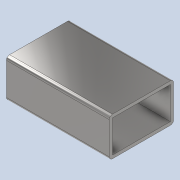
# Autodesk Inventor part: 3in x 5in Steel Rectangular Tubing 8in long
Saved by Autodesk Inventor 2022 (Build 260153000, 153)
## iProperties
Created: 2021-10-11
Part Number: 3in x 5in Steel Rectangular Tubing 8in long
Material: Generic
Document SubType Name: Modeling
Designer: Coy
Density: 1 g/cm^3
Appearance: Galvanized
Author: Coy
Autodesk Inventor part; units mm, degrees
ref_plane "YZ Plane" through (0, 0, 0) normal (1, 0, 0) x (0, 1, 0)
ref_plane "XZ Plane" through (0, 0, 0) normal (0, 1, 0) x (-1, 0, 0)
ref_plane "XY Plane" through (0, 0, 0) normal (0, 0, 1) x (1, 0, 0)
sketch "Sketch1" plane through (0, 0, 0) normal (1, 0, 0) x (0, 1, 0)
  line L0 (6.35, 0) -> (69.85, 0)
  line L1 (76.2, -6.35) -> (76.2, -120.65)
  line L2 (69.85, -127) -> (6.35, -127)
  line L3 (0, -120.65) -> (0, -6.35)
  arc A0 (76.2, -6.35) -> (69.85, 0) centre (69.85, -6.35) ccw
  arc A1 (69.85, -127) -> (76.2, -120.65) centre (69.85, -120.65) ccw
  arc A2 (0, -120.65) -> (6.35, -127) centre (6.35, -120.65) ccw
  arc A3 (6.35, 0) -> (0, -6.35) centre (6.35, -6.35) ccw
  line L4 (69.85, -120.65) -> (69.85, -6.35)
  line L5 (69.85, -6.35) -> (6.35, -6.35)
  line L6 (6.35, -6.35) -> (6.35, -120.65)
  line L7 (6.35, -120.65) -> (69.85, -120.65)
  point P0 (0, 0)
  point P1 (76.2, -127)
  point P2 (76.2, 0)
  point P3 (0, -127)
  dimension "d0" = 76.2
  dimension "d1" = 127
  dimension "d2" = 6.35
  dimension "d3" = 6.35
  dimension "d4" = 6.35
  constraints: 16 end point, 8 point on circle, 8 point on line, 8 tangent, 4 centre point, 4 parallel, 2 equal radius, 2 perpendicular, 1 horizontal, 3 other
  measures "d0" distance of point (76.2, -127) point (0, -127)
  measures "d1" distance of point (76.2, 0) point (76.2, -127)
  measures "d2" radius of A0
  measures "d3" radius of A3
  measures "d4" distance between parallel lines of L1 L4
extrude "Extrusion1" add sketch "Sketch1" against normal blind 203.2
body "Solid1"
